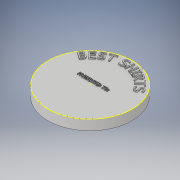
# Autodesk Inventor part: Best Shirts
Saved by Autodesk Inventor 2018.2 (Build 222227000, 227)
## iProperties
Created: 2018-03-07
Part Number: Best Shirts
Material: Generic
Document SubType Name: Modeling
Designer: battin.michael
Density: 1 g/cm^3
Appearance: Default
Author: battin.michael
Autodesk Inventor part; units mm, degrees
ref_plane "YZ Plane" through (0, 0, 0) normal (1, 0, 0) x (0, 1, 0)
ref_plane "XZ Plane" through (0, 0, 0) normal (0, 1, 0) x (-1, 0, 0)
ref_plane "XY Plane" through (0, 0, 0) normal (0, 0, 1) x (1, 0, 0)
sketch "Sketch1" plane through (0, 0, 0) normal (0, 1, 0) x (-1, 0, 0)
  circle A0 centre (0, 0) radius 104.775
  dimension "d0" = 209.55
  constraints: 1 centre point, 1 coincident
  measures "d0" diameter of A0
extrude "Extrusion1" add sketch "Sketch1" along normal blind 25.4
sketch "Sketch2" plane through (0, 25.4, 0) normal (0, 1, 0) x (1, 0, 0)
  circle A0 centre (0, 0) radius 104.775
  spline S0 degree 2 poles (-64.2326, 55.1931) (-62.9995, 54.313) (-61.7794, 52.0259) (-61.7177, 50.8085) knots 0 0 0 1 2 2 2
  spline S1 degree 2 poles (-61.7177, 50.8085) (-61.6636, 49.3537) (-62.5681, 46.7826) (-63.7735, 45.0938) knots 0 0 0 1 2 2 2
  line L0 (-63.7735, 45.0938) -> (-67.16, 40.3492)
  line L1 (-67.16, 40.3492) -> (-83.6992, 52.1542)
  line L2 (-83.6992, 52.1542) -> (-80.571, 56.5369)
  spline S2 degree 2 poles (-80.571, 56.5369) (-79.3082, 58.3061) (-77.8176, 59.9127) (-76.8013, 60.4011) knots 0 0 0 1 2 2 2
  spline S3 degree 2 poles (-76.8013, 60.4011) (-75.6913, 60.9643) (-73.5664, 60.6818) (-72.5209, 59.9356) knots 0 0 0 1 2 2 2
  spline S4 degree 2 poles (-72.5209, 59.9356) (-71.3549, 59.1033) (-70.3854, 56.5501) (-70.6376, 55.0913) knots 0 0 0 1 2 2 2
  line L3 (-70.6376, 55.0913) -> (-70.5571, 55.0339)
  spline S5 degree 2 poles (-70.5571, 55.0339) (-69.1027, 56.2213) (-65.8141, 56.322) (-64.2326, 55.1931) knots 0 0 0 1 2 2 2
  spline S6 degree 2 poles (-65.7746, 52.8343) (-66.7128, 53.5039) (-68.3018, 53.8288) (-69.3046, 53.3307) knots 0 0 0 1 2 2 2
  spline S7 degree 2 poles (-69.3046, 53.3307) (-69.9458, 52.9993) (-70.9867, 51.8811) (-71.7999, 50.7418) knots 0 0 0 1 2 2 2
  line L4 (-71.7999, 50.7418) -> (-73.5792, 48.2489)
  line L5 (-73.5792, 48.2489) -> (-67.4675, 43.8866)
  line L6 (-67.4675, 43.8866) -> (-66.1952, 45.6692)
  spline S8 degree 2 poles (-66.1952, 45.6692) (-65.162, 47.1167) (-64.2438, 48.97) (-64.2135, 49.9194) knots 0 0 0 1 2 2 2
  spline S9 degree 2 poles (-64.2135, 49.9194) (-64.2158, 50.8517) (-64.9034, 52.2124) (-65.7746, 52.8343) knots 0 0 0 1 2 2 2
  spline S10 degree 2 poles (-73.8485, 57.4237) (-74.4383, 57.8446) (-75.6098, 58.0739) (-76.1802, 57.8133) knots 0 0 0 1 2 2 2
  spline S11 degree 2 poles (-76.1802, 57.8133) (-76.8577, 57.4877) (-77.9197, 56.2833) (-78.752, 55.1172) knots 0 0 0 1 2 2 2
  line L7 (-78.752, 55.1172) -> (-80.2539, 53.0129)
  line L8 (-80.2539, 53.0129) -> (-75.4154, 49.5595)
  line L9 (-75.4154, 49.5595) -> (-73.6361, 52.0524)
  spline S12 degree 2 poles (-73.6361, 52.0524) (-72.8995, 53.0844) (-72.4156, 54.2159) (-72.3775, 54.9778) knots 0 0 0 1 2 2 2
  spline S13 degree 2 poles (-72.3775, 54.9778) (-72.3357, 55.7167) (-73.0712, 56.8688) (-73.8485, 57.4237) knots 0 0 0 1 2 2 2
  line L10 (-57.2472, 53.4467) -> (-71.0363, 68.372)
  line L11 (-71.0363, 68.372) -> (-61.699, 76.9986)
  line L12 (-61.699, 76.9986) -> (-60.0675, 75.2327)
  line L13 (-60.0675, 75.2327) -> (-67.4213, 68.4387)
  line L14 (-67.4213, 68.4387) -> (-63.6444, 64.3506)
  line L15 (-63.6444, 64.3506) -> (-56.7865, 70.6864)
  line L16 (-56.7865, 70.6864) -> (-55.155, 68.9205)
  line L17 (-55.155, 68.9205) -> (-62.0129, 62.5847)
  line L18 (-62.0129, 62.5847) -> (-56.8951, 57.0452)
  line L19 (-56.8951, 57.0452) -> (-49.5413, 63.8392)
  line L20 (-49.5413, 63.8392) -> (-47.9099, 62.0733)
  line L21 (-47.9099, 62.0733) -> (-57.2472, 53.4467)
  spline S14 degree 2 poles (-40.455, 66.3877) (-42.3401, 65.2409) (-45.4642, 64.4197) (-46.9742, 64.2721) knots 0 0 0 1 2 2 2
  line L22 (-46.9742, 64.2721) -> (-48.7372, 67.1701)
  line L23 (-48.7372, 67.1701) -> (-48.5684, 67.2728)
  spline S15 degree 2 poles (-48.5684, 67.2728) (-46.7784, 66.8969) (-43.1756, 67.4696) (-41.8391, 68.2827) knots 0 0 0 1 2 2 2
  spline S16 degree 2 poles (-41.8391, 68.2827) (-39.9259, 69.4466) (-38.9375, 72.2259) (-39.7334, 73.5342) knots 0 0 0 1 2 2 2
  spline S17 degree 2 poles (-39.7334, 73.5342) (-40.3668, 74.5753) (-42.1811, 75.2448) (-43.4893, 74.8922) knots 0 0 0 1 2 2 2
  spline S18 degree 2 poles (-43.4893, 74.8922) (-44.4281, 74.6295) (-45.9529, 74.1259) (-47.1058, 73.7715) knots 0 0 0 1 2 2 2
  spline S19 degree 2 poles (-47.1058, 73.7715) (-48.1516, 73.4629) (-50.0089, 73.316) (-50.9085, 73.559) knots 0 0 0 1 2 2 2
  spline S20 degree 2 poles (-50.9085, 73.559) (-51.794, 73.8106) (-53.3262, 74.9986) (-53.9425, 76.0115) knots 0 0 0 1 2 2 2
  spline S21 degree 2 poles (-53.9425, 76.0115) (-55.2262, 78.1217) (-53.6717, 82.9801) (-51.1253, 84.5292) knots 0 0 0 1 2 2 2
  spline S22 degree 2 poles (-51.1253, 84.5292) (-49.6623, 85.4193) (-46.7229, 86.4172) (-45.2777, 86.5447) knots 0 0 0 1 2 2 2
  line L24 (-45.2777, 86.5447) -> (-43.6003, 83.7874)
  line L25 (-43.6003, 83.7874) -> (-43.7691, 83.6847)
  spline S23 degree 2 poles (-43.7691, 83.6847) (-45.0613, 83.9394) (-48.3344, 83.4901) (-49.7553, 82.6257) knots 0 0 0 1 2 2 2
  spline S24 degree 2 poles (-49.7553, 82.6257) (-51.3591, 81.65) (-52.4269, 78.938) (-51.6823, 77.7141) knots 0 0 0 1 2 2 2
  spline S25 degree 2 poles (-51.6823, 77.7141) (-51.0148, 76.6168) (-49.0512, 76.0188) (-47.7742, 76.391) knots 0 0 0 1 2 2 2
  spline S26 degree 2 poles (-47.7742, 76.391) (-46.9228, 76.6391) (-44.4904, 77.4249) (-43.6587, 77.6418) knots 0 0 0 1 2 2 2
  spline S27 degree 2 poles (-43.6587, 77.6418) (-41.5382, 78.1801) (-38.5346, 76.9813) (-37.5503, 75.3635) knots 0 0 0 1 2 2 2
  spline S28 degree 2 poles (-37.5503, 75.3635) (-36.9256, 74.3365) (-36.5574, 71.8621) (-36.8837, 70.7191) knots 0 0 0 1 2 2 2
  spline S29 degree 2 poles (-36.8837, 70.7191) (-37.2515, 69.4545) (-38.8653, 67.3548) (-40.455, 66.3877) knots 0 0 0 1 2 2 2
  line L26 (-27.5594, 73.094) -> (-33.5858, 89.9659)
  line L27 (-33.5858, 89.9659) -> (-40.0058, 87.6728)
  line L28 (-40.0058, 87.6728) -> (-40.8145, 89.9368)
  line L29 (-40.8145, 89.9368) -> (-25.4313, 95.4315)
  line L30 (-25.4313, 95.4315) -> (-24.6226, 93.1674)
  line L31 (-24.6226, 93.1674) -> (-31.0426, 90.8743)
  line L32 (-31.0426, 90.8743) -> (-25.0162, 74.0024)
  line L33 (-25.0162, 74.0024) -> (-27.5594, 73.094)
  spline S30 degree 2 poles (-2.2308, 77.7107) (-4.4365, 77.6491) (-7.5568, 78.4843) (-8.9414, 79.1045) knots 0 0 0 1 2 2 2
  line L34 (-8.9414, 79.1045) -> (-9.0363, 82.4953)
  line L35 (-9.0363, 82.4953) -> (-8.8387, 82.5009)
  spline S31 degree 2 poles (-8.8387, 82.5009) (-7.4705, 81.2872) (-4.0574, 79.9989) (-2.4937, 80.0426) knots 0 0 0 1 2 2 2
  spline S32 degree 2 poles (-2.4937, 80.0426) (-0.2551, 80.1052) (1.9809, 82.0292) (1.9381, 83.56) knots 0 0 0 1 2 2 2
  spline S33 degree 2 poles (1.9381, 83.56) (1.904, 84.7781) (0.6601, 86.2588) (-0.6509, 86.601) knots 0 0 0 1 2 2 2
  spline S34 degree 2 poles (-0.6509, 86.601) (-1.5965, 86.8382) (-3.1704, 87.1566) (-4.3473, 87.4202) knots 0 0 0 1 2 2 2
  spline S35 degree 2 poles (-4.3473, 87.4202) (-5.4086, 87.6705) (-7.0946, 88.4635) (-7.7554, 89.1204) knots 0 0 0 1 2 2 2
  spline S36 degree 2 poles (-7.7554, 89.1204) (-8.3998, 89.7778) (-9.1417, 91.5691) (-9.1749, 92.7543) knots 0 0 0 1 2 2 2
  spline S37 degree 2 poles (-9.1749, 92.7543) (-9.2439, 95.2233) (-5.4856, 98.6725) (-2.5063, 98.7558) knots 0 0 0 1 2 2 2
  spline S38 degree 2 poles (-2.5063, 98.7558) (-0.7945, 98.8037) (2.2531, 98.2135) (3.5714, 97.6079) knots 0 0 0 1 2 2 2
  line L36 (3.5714, 97.6079) -> (3.6617, 94.3817)
  line L37 (3.6617, 94.3817) -> (3.4641, 94.3762)
  spline S39 degree 2 poles (3.4641, 94.3762) (2.4681, 95.2379) (-0.5974, 96.47) (-2.2599, 96.4235) knots 0 0 0 1 2 2 2
  spline S40 degree 2 poles (-2.2599, 96.4235) (-4.1364, 96.371) (-6.408, 94.5449) (-6.368, 93.1128) knots 0 0 0 1 2 2 2
  spline S41 degree 2 poles (-6.368, 93.1128) (-6.3321, 91.8289) (-4.9231, 90.3363) (-3.6295, 90.0265) knots 0 0 0 1 2 2 2
  spline S42 degree 2 poles (-3.6295, 90.0265) (-2.7671, 89.82) (-0.265, 89.297) (0.5649, 89.0731) knots 0 0 0 1 2 2 2
  spline S43 degree 2 poles (0.5649, 89.0731) (2.6733, 88.4896) (4.6879, 85.9596) (4.7408, 84.0667) knots 0 0 0 1 2 2 2
  spline S44 degree 2 poles (4.7408, 84.0667) (4.7744, 82.8651) (3.8677, 80.5335) (3.0179, 79.7025) knots 0 0 0 1 2 2 2
  spline S45 degree 2 poles (3.0179, 79.7025) (2.0716, 78.7865) (-0.3708, 77.7628) (-2.2308, 77.7107) knots 0 0 0 1 2 2 2
  line L38 (22.1122, 75.2719) -> (19.461, 75.7861)
  line L39 (19.461, 75.7861) -> (21.3546, 85.5501)
  line L40 (21.3546, 85.5501) -> (12.1725, 87.3308)
  line L41 (12.1725, 87.3308) -> (10.279, 77.5668)
  line L42 (10.279, 77.5668) -> (7.6278, 78.0809)
  line L43 (7.6278, 78.0809) -> (11.4964, 98.0293)
  line L44 (11.4964, 98.0293) -> (14.1476, 97.5151)
  line L45 (14.1476, 97.5151) -> (12.6302, 89.691)
  line L46 (12.6302, 89.691) -> (21.8123, 87.9103)
  line L47 (21.8123, 87.9103) -> (23.3296, 95.7344)
  line L48 (23.3296, 95.7344) -> (25.9808, 95.2203)
  line L49 (25.9808, 95.2203) -> (22.1122, 75.2719)
  line L50 (32.5045, 71.1286) -> (25.1902, 74.0365)
  line L51 (25.1902, 74.0365) -> (25.9567, 75.9645)
  line L52 (25.9567, 75.9645) -> (28.3591, 75.0094)
  line L53 (28.3591, 75.0094) -> (34.3331, 90.0358)
  line L54 (34.3331, 90.0358) -> (31.9307, 90.9909)
  line L55 (31.9307, 90.9909) -> (32.6972, 92.9189)
  line L56 (32.6972, 92.9189) -> (40.0115, 90.011)
  line L57 (40.0115, 90.011) -> (39.245, 88.083)
  line L58 (39.245, 88.083) -> (36.8426, 89.0381)
  line L59 (36.8426, 89.0381) -> (30.8686, 74.0117)
  line L60 (30.8686, 74.0117) -> (33.271, 73.0566)
  line L61 (33.271, 73.0566) -> (32.5045, 71.1286)
  line L62 (48.939, 61.5502) -> (45.9592, 63.4002)
  line L63 (45.9592, 63.4002) -> (44.7675, 73.6565)
  line L64 (44.7675, 73.6565) -> (42.1373, 75.2894)
  line L65 (42.1373, 75.2894) -> (37.8729, 68.4202)
  line L66 (37.8729, 68.4202) -> (35.5785, 69.8446)
  line L67 (35.5785, 69.8446) -> (46.2961, 87.1084)
  line L68 (46.2961, 87.1084) -> (50.7449, 84.3465)
  spline S46 degree 2 poles (50.7449, 84.3465) (52.2279, 83.4258) (54.0287, 81.8621) (54.5732, 80.71) knots 0 0 0 1 2 2 2
  spline S47 degree 2 poles (54.5732, 80.71) (55.1178, 79.5578) (55.0293, 77.0737) (54.1869, 75.7167) knots 0 0 0 1 2 2 2
  spline S48 degree 2 poles (54.1869, 75.7167) (53.0144, 73.8281) (49.4943, 72.4664) (47.4614, 72.8757) knots 0 0 0 1 2 2 2
  line L69 (47.4614, 72.8757) -> (48.939, 61.5502)
  spline S49 degree 2 poles (51.6816, 77.02) (52.1506, 77.7755) (52.3399, 79.2667) (52.0148, 79.9918) knots 0 0 0 1 2 2 2
  spline S50 degree 2 poles (52.0148, 79.9918) (51.7249, 80.6176) (50.5888, 81.6911) (49.6375, 82.2817) knots 0 0 0 1 2 2 2
  line L70 (49.6375, 82.2817) -> (47.3571, 83.6974)
  line L71 (47.3571, 83.6974) -> (43.3272, 77.206)
  line L72 (43.3272, 77.206) -> (45.3418, 75.9553)
  spline S51 degree 2 poles (45.3418, 75.9553) (46.3351, 75.3387) (48.1331, 74.707) (49.0174, 74.9139) knots 0 0 0 1 2 2 2
  spline S52 degree 2 poles (49.0174, 74.9139) (49.8163, 75.0769) (51.1258, 76.1246) (51.6816, 77.02) knots 0 0 0 1 2 2 2
  line L73 (53.4089, 57.0066) -> (65.8849, 69.8645)
  line L74 (65.8849, 69.8645) -> (60.9922, 74.6118)
  line L75 (60.9922, 74.6118) -> (62.6664, 76.3373)
  line L76 (62.6664, 76.3373) -> (74.3898, 64.9621)
  line L77 (74.3898, 64.9621) -> (72.7157, 63.2367)
  line L78 (72.7157, 63.2367) -> (67.823, 67.984)
  line L79 (67.823, 67.984) -> (55.347, 55.126)
  line L80 (55.347, 55.126) -> (53.4089, 57.0066)
  spline S53 degree 2 poles (64.2632, 43.7513) (63.0228, 45.5762) (62.0451, 48.6549) (61.8215, 50.1555) knots 0 0 0 1 2 2 2
  line L81 (61.8215, 50.1555) -> (64.6269, 52.0624)
  line L82 (64.6269, 52.0624) -> (64.738, 51.899)
  spline S54 degree 2 poles (64.738, 51.899) (64.4528, 50.0923) (65.2065, 46.523) (66.086, 45.2292) knots 0 0 0 1 2 2 2
  spline S55 degree 2 poles (66.086, 45.2292) (67.3449, 43.3771) (70.1705, 42.5301) (71.437, 43.391) knots 0 0 0 1 2 2 2
  spline S56 degree 2 poles (71.437, 43.391) (72.4448, 44.076) (73.0219, 45.9218) (72.6039, 47.2106) knots 0 0 0 1 2 2 2
  spline S57 degree 2 poles (72.6039, 47.2106) (72.2941, 48.135) (71.7143, 49.6324) (71.3022, 50.7659) knots 0 0 0 1 2 2 2
  spline S58 degree 2 poles (71.3022, 50.7659) (70.9413, 51.7949) (70.7009, 53.6425) (70.8982, 54.5531) knots 0 0 0 1 2 2 2
  spline S59 degree 2 poles (70.8982, 54.5531) (71.1048, 55.4501) (72.2141, 57.0404) (73.1946, 57.7069) knots 0 0 0 1 2 2 2
  spline S60 degree 2 poles (73.1946, 57.7069) (75.2374, 59.0954) (80.1681, 57.7878) (81.8436, 55.3229) knots 0 0 0 1 2 2 2
  spline S61 degree 2 poles (81.8436, 55.3229) (82.8063, 53.9066) (83.9512, 51.0212) (84.1514, 49.5843) knots 0 0 0 1 2 2 2
  line L83 (84.1514, 49.5843) -> (81.4821, 47.77)
  line L84 (81.4821, 47.77) -> (81.3711, 47.9334)
  spline S62 degree 2 poles (81.3711, 47.9334) (81.5603, 49.2368) (80.9465, 52.4831) (80.0116, 53.8586) knots 0 0 0 1 2 2 2
  spline S63 degree 2 poles (80.0116, 53.8586) (78.9563, 55.4111) (76.1939, 56.3408) (75.009, 55.5355) knots 0 0 0 1 2 2 2
  spline S64 degree 2 poles (75.009, 55.5355) (73.9468, 54.8134) (73.4486, 52.8222) (73.8847, 51.5656) knots 0 0 0 1 2 2 2
  spline S65 degree 2 poles (73.8847, 51.5656) (74.1754, 50.7278) (75.0829, 48.3382) (75.3414, 47.5184) knots 0 0 0 1 2 2 2
  spline S66 degree 2 poles (75.3414, 47.5184) (75.986, 45.4278) (74.9402, 42.3675) (73.374, 41.3029) knots 0 0 0 1 2 2 2
  spline S67 degree 2 poles (73.374, 41.3029) (72.3799, 40.6272) (69.9271, 40.1347) (68.7692, 40.4029) knots 0 0 0 1 2 2 2
  spline S68 degree 2 poles (68.7692, 40.4029) (67.4876, 40.7065) (65.3092, 42.2124) (64.2632, 43.7513) knots 0 0 0 1 2 2 2
  constraints: 1 centre point, 1 coincident, 1 other
extrude "Extrusion2" add sketch "Sketch2" along normal blind 5.08 contours S0 S1 L0 L1 L2 S2 S3 S4 L3 S5 | L10 L11 L12 L13 L14 L15 L16 L17 L18 L19 L20 L21 | S14 L22 L23 S15 S16 S17 S18 S19 S20 S21 S22 L24 L25 S23 S24 S25 S26 S27 S28 S29 | L26 L27 L28 L29 L30 L31 L32 L33 | S30 L34 L35 S31 S32 S33 S34 S35 S36 S37 S38 L36 L37 S39 S40 S41 S42 S43 S44 S45 | L38 L39 L40 L41 L42 L43 L44 L45 L46 L47 L48 L49 | L50 L51 L52 L53 L54 L55 L56 L57 L58 L59 L60 L61 | L62 L63 L64 L65 L66 L67 L68 S46 S47 S48 L69 | L73 L74 L75 L76 L77 L78 L79 L80 | S53 L81 L82 S54 S55 S56 S57 S58 S59 S60 S61 L83 L84 S62 S63 S64 S65 S66 S67 S68
sketch "Sketch3" plane through (0, 25.4, 0) normal (0, 1, 0) x (1, 0, 0)
  circle A0 centre (0, 0) radius 104.775
  constraints: 1 centre point, 1 coincident
extrude "Extrusion3" add sketch "Sketch3" along normal blind 2.54
sketch "Sketch4" plane through (0, 0, 0) normal (0, -1, 0) x (1, 0, 0)
  circle A0 centre (0, 0) radius 104.775
  constraints: 1 centre point, 1 coincident
extrude "Extrusion4" cut sketch "Sketch4" against normal blind 2.54
sketch "Sketch5" plane through (0, 27.94, 0) normal (0, 1, 0) x (1, 0, 0)
  circle A0 centre (0, 0) radius 104.775 projected
  circle A1 centre (0, 0) radius 104.775 projected
sketch "Sketch6" plane through (0, 27.94, 0) normal (0, 1, 0) x (1, 0, 0)
  circle A0 centre (0, 0) radius 104.775 projected
  spline S0 degree 2 poles (-32.6567, 10.8618) (-32.6567, 10.3678) (-33.0087, 9.4786) (-33.3236, 9.1698) knots 0 0 0 1 2 2 2
  spline S1 degree 2 poles (-33.3236, 9.1698) (-33.7188, 8.7808) (-34.7871, 8.3794) (-35.6022, 8.3794) knots 0 0 0 1 2 2 2
  line L0 (-35.6022, 8.3794) -> (-36.4605, 8.3794)
  line L1 (-36.4605, 8.3794) -> (-36.4605, 5.5389)
  line L2 (-36.4605, 5.5389) -> (-37.4732, 5.5389)
  line L3 (-37.4732, 5.5389) -> (-37.4732, 13.1589)
  line L4 (-37.4732, 13.1589) -> (-35.559, 13.1589)
  spline S2 degree 2 poles (-35.559, 13.1589) (-34.8797, 13.1589) (-33.9288, 12.9366) (-33.5644, 12.6834) knots 0 0 0 1 2 2 2
  spline S3 degree 2 poles (-33.5644, 12.6834) (-33.1384, 12.3932) (-32.6567, 11.4978) (-32.6567, 10.8618) knots 0 0 0 1 2 2 2
  spline S4 degree 2 poles (-33.7126, 10.8309) (-33.7126, 11.2261) (-33.9843, 11.8066) (-34.2622, 11.9918) knots 0 0 0 1 2 2 2
  spline S5 degree 2 poles (-34.2622, 11.9918) (-34.503, 12.1524) (-35.1452, 12.2821) (-35.6207, 12.2821) knots 0 0 0 1 2 2 2
  line L5 (-35.6207, 12.2821) -> (-36.4605, 12.2821)
  line L6 (-36.4605, 12.2821) -> (-36.4605, 9.2439)
  line L7 (-36.4605, 9.2439) -> (-35.7689, 9.2439)
  spline S6 degree 2 poles (-35.7689, 9.2439) (-35.1514, 9.2439) (-34.3919, 9.4415) (-34.1449, 9.7009) knots 0 0 0 1 2 2 2
  spline S7 degree 2 poles (-34.1449, 9.7009) (-33.9164, 9.9294) (-33.7126, 10.4666) (-33.7126, 10.8309) knots 0 0 0 1 2 2 2
  line L8 (-25.7962, 5.5389) -> (-27.1115, 5.5389)
  line L9 (-27.1115, 5.5389) -> (-29.5198, 8.5709)
  line L10 (-29.5198, 8.5709) -> (-30.6807, 8.5709)
  line L11 (-30.6807, 8.5709) -> (-30.6807, 5.5389)
  line L12 (-30.6807, 5.5389) -> (-31.6934, 5.5389)
  line L13 (-31.6934, 5.5389) -> (-31.6934, 13.1589)
  line L14 (-31.6934, 13.1589) -> (-29.7297, 13.1589)
  spline S8 degree 2 poles (-29.7297, 13.1589) (-29.0752, 13.1589) (-28.1921, 13.0169) (-27.7908, 12.7575) knots 0 0 0 1 2 2 2
  spline S9 degree 2 poles (-27.7908, 12.7575) (-27.3894, 12.4982) (-26.9263, 11.6893) (-26.9263, 11.0903) knots 0 0 0 1 2 2 2
  spline S10 degree 2 poles (-26.9263, 11.0903) (-26.9263, 10.2567) (-27.7784, 9.1266) (-28.5071, 8.8549) knots 0 0 0 1 2 2 2
  line L15 (-28.5071, 8.8549) -> (-25.7962, 5.5389)
  spline S11 degree 2 poles (-27.9822, 11.01) (-27.9822, 11.3435) (-28.2168, 11.856) (-28.4638, 12.0227) knots 0 0 0 1 2 2 2
  spline S12 degree 2 poles (-28.4638, 12.0227) (-28.68, 12.1647) (-29.2543, 12.2821) (-29.6742, 12.2821) knots 0 0 0 1 2 2 2
  line L16 (-29.6742, 12.2821) -> (-30.6807, 12.2821)
  line L17 (-30.6807, 12.2821) -> (-30.6807, 9.4168)
  line L18 (-30.6807, 9.4168) -> (-29.7915, 9.4168)
  spline S13 degree 2 poles (-29.7915, 9.4168) (-29.3531, 9.4168) (-28.6553, 9.5712) (-28.4144, 9.8121) knots 0 0 0 1 2 2 2
  spline S14 degree 2 poles (-28.4144, 9.8121) (-28.1921, 10.022) (-27.9822, 10.6148) (-27.9822, 11.01) knots 0 0 0 1 2 2 2
  line L19 (-25.1911, 5.5389) -> (-25.1911, 13.1589)
  line L20 (-25.1911, 13.1589) -> (-20.4239, 13.1589)
  line L21 (-20.4239, 13.1589) -> (-20.4239, 12.2574)
  line L22 (-20.4239, 12.2574) -> (-24.1784, 12.2574)
  line L23 (-24.1784, 12.2574) -> (-24.1784, 10.1702)
  line L24 (-24.1784, 10.1702) -> (-20.6771, 10.1702)
  line L25 (-20.6771, 10.1702) -> (-20.6771, 9.2686)
  line L26 (-20.6771, 9.2686) -> (-24.1784, 9.2686)
  line L27 (-24.1784, 9.2686) -> (-24.1784, 6.4405)
  line L28 (-24.1784, 6.4405) -> (-20.4239, 6.4405)
  line L29 (-20.4239, 6.4405) -> (-20.4239, 5.5389)
  line L30 (-20.4239, 5.5389) -> (-25.1911, 5.5389)
  spline S15 degree 2 poles (-17.1882, 5.4031) (-18.0157, 5.4031) (-19.1766, 5.7489) (-19.6891, 5.9959) knots 0 0 0 1 2 2 2
  line L31 (-19.6891, 5.9959) -> (-19.6891, 7.2679)
  line L32 (-19.6891, 7.2679) -> (-19.615, 7.2679)
  spline S16 degree 2 poles (-19.615, 7.2679) (-19.1148, 6.7986) (-17.849, 6.2799) (-17.2623, 6.2799) knots 0 0 0 1 2 2 2
  spline S17 degree 2 poles (-17.2623, 6.2799) (-16.4225, 6.2799) (-15.5642, 6.9777) (-15.5642, 7.552) knots 0 0 0 1 2 2 2
  spline S18 degree 2 poles (-15.5642, 7.552) (-15.5642, 8.0089) (-16.015, 8.577) (-16.5028, 8.7191) knots 0 0 0 1 2 2 2
  spline S19 degree 2 poles (-16.5028, 8.7191) (-16.8548, 8.8179) (-17.4414, 8.9537) (-17.8798, 9.0649) knots 0 0 0 1 2 2 2
  spline S20 degree 2 poles (-17.8798, 9.0649) (-18.275, 9.1698) (-18.8987, 9.4848) (-19.1395, 9.738) knots 0 0 0 1 2 2 2
  spline S21 degree 2 poles (-19.1395, 9.738) (-19.3742, 9.9911) (-19.6335, 10.6704) (-19.6335, 11.115) knots 0 0 0 1 2 2 2
  spline S22 degree 2 poles (-19.6335, 11.115) (-19.6335, 12.0412) (-18.1886, 13.2948) (-17.0709, 13.2948) knots 0 0 0 1 2 2 2
  spline S23 degree 2 poles (-17.0709, 13.2948) (-16.4287, 13.2948) (-15.2925, 13.0416) (-14.8047, 12.8008) knots 0 0 0 1 2 2 2
  line L33 (-14.8047, 12.8008) -> (-14.8047, 11.5905)
  line L34 (-14.8047, 11.5905) -> (-14.8788, 11.5905)
  spline S24 degree 2 poles (-14.8788, 11.5905) (-15.2431, 11.9239) (-16.3793, 12.4179) (-17.003, 12.4179) knots 0 0 0 1 2 2 2
  spline S25 degree 2 poles (-17.003, 12.4179) (-17.7069, 12.4179) (-18.5776, 11.7572) (-18.5776, 11.22) knots 0 0 0 1 2 2 2
  spline S26 degree 2 poles (-18.5776, 11.22) (-18.5776, 10.7383) (-18.0651, 10.164) (-17.5834, 10.0344) knots 0 0 0 1 2 2 2
  spline S27 degree 2 poles (-17.5834, 10.0344) (-17.2623, 9.9479) (-16.3299, 9.7256) (-16.0211, 9.633) knots 0 0 0 1 2 2 2
  spline S28 degree 2 poles (-16.0211, 9.633) (-15.2369, 9.3921) (-14.5083, 8.4227) (-14.5083, 7.7125) knots 0 0 0 1 2 2 2
  spline S29 degree 2 poles (-14.5083, 7.7125) (-14.5083, 7.2618) (-14.8726, 6.3973) (-15.1999, 6.0947) knots 0 0 0 1 2 2 2
  spline S30 degree 2 poles (-15.1999, 6.0947) (-15.5642, 5.7612) (-16.4904, 5.4031) (-17.1882, 5.4031) knots 0 0 0 1 2 2 2
  line L35 (-13.477, 5.5389) -> (-13.477, 13.1589)
  line L36 (-13.477, 13.1589) -> (-8.7099, 13.1589)
  line L37 (-8.7099, 13.1589) -> (-8.7099, 12.2574)
  line L38 (-8.7099, 12.2574) -> (-12.4643, 12.2574)
  line L39 (-12.4643, 12.2574) -> (-12.4643, 10.1702)
  line L40 (-12.4643, 10.1702) -> (-8.9631, 10.1702)
  line L41 (-8.9631, 10.1702) -> (-8.9631, 9.2686)
  line L42 (-8.9631, 9.2686) -> (-12.4643, 9.2686)
  line L43 (-12.4643, 9.2686) -> (-12.4643, 6.4405)
  line L44 (-12.4643, 6.4405) -> (-8.7099, 6.4405)
  line L45 (-8.7099, 6.4405) -> (-8.7099, 5.5389)
  line L46 (-8.7099, 5.5389) -> (-13.477, 5.5389)
  line L47 (-2.1458, 5.5389) -> (-3.282, 5.5389)
  line L48 (-3.282, 5.5389) -> (-6.6536, 12.1092)
  line L49 (-6.6536, 12.1092) -> (-6.6536, 5.5389)
  line L50 (-6.6536, 5.5389) -> (-7.5984, 5.5389)
  line L51 (-7.5984, 5.5389) -> (-7.5984, 13.1589)
  line L52 (-7.5984, 13.1589) -> (-6.1596, 13.1589)
  line L53 (-6.1596, 13.1589) -> (-3.0906, 7.1259)
  line L54 (-3.0906, 7.1259) -> (-3.0906, 13.1589)
  line L55 (-3.0906, 13.1589) -> (-2.1458, 13.1589)
  line L56 (-2.1458, 13.1589) -> (-2.1458, 5.5389)
  line L57 (1.1763, 5.5389) -> (1.1763, 12.2574)
  line L58 (1.1763, 12.2574) -> (-1.3801, 12.2574)
  line L59 (-1.3801, 12.2574) -> (-1.3801, 13.1589)
  line L60 (-1.3801, 13.1589) -> (4.7455, 13.1589)
  line L61 (4.7455, 13.1589) -> (4.7455, 12.2574)
  line L62 (4.7455, 12.2574) -> (2.1891, 12.2574)
  line L63 (2.1891, 12.2574) -> (2.1891, 5.5389)
  line L64 (2.1891, 5.5389) -> (1.1763, 5.5389)
  line L65 (5.5174, 5.5389) -> (5.5174, 13.1589)
  line L66 (5.5174, 13.1589) -> (10.2845, 13.1589)
  line L67 (10.2845, 13.1589) -> (10.2845, 12.2574)
  line L68 (10.2845, 12.2574) -> (6.5301, 12.2574)
  line L69 (6.5301, 12.2574) -> (6.5301, 10.1702)
  line L70 (6.5301, 10.1702) -> (10.0314, 10.1702)
  line L71 (10.0314, 10.1702) -> (10.0314, 9.2686)
  line L72 (10.0314, 9.2686) -> (6.5301, 9.2686)
  line L73 (6.5301, 9.2686) -> (6.5301, 6.4405)
  line L74 (6.5301, 6.4405) -> (10.2845, 6.4405)
  line L75 (10.2845, 6.4405) -> (10.2845, 5.5389)
  line L76 (10.2845, 5.5389) -> (5.5174, 5.5389)
  spline S31 degree 2 poles (17.4044, 9.3427) (17.4044, 8.2992) (16.5584, 6.6196) (15.8482, 6.1503) knots 0 0 0 1 2 2 2
  spline S32 degree 2 poles (15.8482, 6.1503) (15.2678, 5.7859) (14.076, 5.5389) (13.1498, 5.5389) knots 0 0 0 1 2 2 2
  line L77 (13.1498, 5.5389) -> (11.396, 5.5389)
  line L78 (11.396, 5.5389) -> (11.396, 13.1589)
  line L79 (11.396, 13.1589) -> (13.1312, 13.1589)
  spline S33 degree 2 poles (13.1312, 13.1589) (14.2057, 13.1589) (15.4283, 12.8378) (15.8606, 12.5538) knots 0 0 0 1 2 2 2
  spline S34 degree 2 poles (15.8606, 12.5538) (16.5954, 12.0659) (17.4044, 10.4543) (17.4044, 9.3427) knots 0 0 0 1 2 2 2
  spline S35 degree 2 poles (16.3484, 9.3551) (16.3484, 10.232) (15.768, 11.4731) (15.1937, 11.8251) knots 0 0 0 1 2 2 2
  spline S36 degree 2 poles (15.1937, 11.8251) (14.7861, 12.0659) (13.8661, 12.2821) (13.1806, 12.2821) knots 0 0 0 1 2 2 2
  line L80 (13.1806, 12.2821) -> (12.4087, 12.2821)
  line L81 (12.4087, 12.2821) -> (12.4087, 6.4158)
  line L82 (12.4087, 6.4158) -> (13.1806, 6.4158)
  spline S37 degree 2 poles (13.1806, 6.4158) (13.8537, 6.4158) (14.8726, 6.6319) (15.2863, 6.9221) knots 0 0 0 1 2 2 2
  spline S38 degree 2 poles (15.2863, 6.9221) (15.8174, 7.2803) (16.3484, 8.4659) (16.3484, 9.3551) knots 0 0 0 1 2 2 2
  line L83 (23.5547, 5.5389) -> (23.5547, 12.2574)
  line L84 (23.5547, 12.2574) -> (20.9982, 12.2574)
  line L85 (20.9982, 12.2574) -> (20.9982, 13.1589)
  line L86 (20.9982, 13.1589) -> (27.1239, 13.1589)
  line L87 (27.1239, 13.1589) -> (27.1239, 12.2574)
  line L88 (27.1239, 12.2574) -> (24.5674, 12.2574)
  line L89 (24.5674, 12.2574) -> (24.5674, 5.5389)
  line L90 (24.5674, 5.5389) -> (23.5547, 5.5389)
  spline S39 degree 2 poles (33.2866, 12.2882) (33.7188, 11.7819) (34.2005, 10.2999) (34.2005, 9.3489) knots 0 0 0 1 2 2 2
  spline S40 degree 2 poles (34.2005, 9.3489) (34.2005, 8.4227) (33.7312, 6.9221) (33.2866, 6.4158) knots 0 0 0 1 2 2 2
  spline S41 degree 2 poles (33.2866, 6.4158) (32.8173, 5.8847) (31.5761, 5.3784) (30.8289, 5.3784) knots 0 0 0 1 2 2 2
  spline S42 degree 2 poles (30.8289, 5.3784) (30.057, 5.3784) (28.822, 5.9033) (28.3712, 6.4158) knots 0 0 0 1 2 2 2
  spline S43 degree 2 poles (28.3712, 6.4158) (27.9328, 6.9221) (27.4635, 8.4103) (27.4635, 9.3489) knots 0 0 0 1 2 2 2
  spline S44 degree 2 poles (27.4635, 9.3489) (27.4635, 10.3061) (27.939, 11.7634) (28.3774, 12.2882) knots 0 0 0 1 2 2 2
  spline S45 degree 2 poles (28.3774, 12.2882) (28.822, 12.7946) (30.0632, 13.3195) (30.8289, 13.3195) knots 0 0 0 1 2 2 2
  spline S46 degree 2 poles (30.8289, 13.3195) (31.6069, 13.3195) (32.8543, 12.7761) (33.2866, 12.2882) knots 0 0 0 1 2 2 2
  spline S47 degree 2 poles (33.1445, 9.3489) (33.1445, 10.1023) (32.8173, 11.2694) (32.5209, 11.6522) knots 0 0 0 1 2 2 2
  spline S48 degree 2 poles (32.5209, 11.6522) (32.2183, 12.0474) (31.3661, 12.4426) (30.8351, 12.4426) knots 0 0 0 1 2 2 2
  spline S49 degree 2 poles (30.8351, 12.4426) (30.2855, 12.4426) (29.458, 12.0598) (29.1431, 11.6522) knots 0 0 0 1 2 2 2
  spline S50 degree 2 poles (29.1431, 11.6522) (28.8405, 11.2632) (28.5194, 10.0899) (28.5194, 9.3489) knots 0 0 0 1 2 2 2
  spline S51 degree 2 poles (28.5194, 9.3489) (28.5194, 7.8484) (29.7791, 6.2552) (30.8351, 6.2552) knots 0 0 0 1 2 2 2
  spline S52 degree 2 poles (30.8351, 6.2552) (31.891, 6.2552) (33.1445, 7.8484) (33.1445, 9.3489) knots 0 0 0 1 2 2 2
  line L91 (37.0039, 5.5389) -> (35.7813, 5.5389)
  line L92 (35.7813, 5.5389) -> (35.7813, 6.9962)
  line L93 (35.7813, 6.9962) -> (37.0039, 6.9962)
  line L94 (37.0039, 6.9962) -> (37.0039, 5.5389)
  line L95 (37.0039, 9.7997) -> (35.7813, 9.7997)
  line L96 (35.7813, 9.7997) -> (35.7813, 11.257)
  line L97 (35.7813, 11.257) -> (37.0039, 11.257)
  line L98 (37.0039, 11.257) -> (37.0039, 9.7997)
  point P0 (-38.2451, 5.5389)
  constraints: 1 other
extrude "Extrusion5" add sketch "Sketch6" along normal blind 2.54 contours S0 S1 L0 L1 L2 L3 L4 S2 S3 | L8 L9 L10 L11 L12 L13 L14 S8 S9 S10 L15 | L19 L20 L21 L22 L23 L24 L25 L26 L27 L28 L29 L30 | S15 L31 L32 S16 S17 S18 S19 S20 S21 S22 S23 L33 L34 S24 S25 S26 S27 S28 S29 S30 | L35 L36 L37 L38 L39 L40 L41 L42 L43 L44 L45 L46 | L47 L48 L49 L50 L51 L52 L53 L54 L55 L56 | L57 L58 L59 L60 L61 L62 L63 L64 | L65 L66 L67 L68 L69 L70 L71 L72 L73 L74 L75 L76 | S31 S32 L77 L78 L79 S33 S34 | L83 L84 L85 L86 L87 L88 L89 L90 | S39 S40 S41 S42 S43 S44 S45 S46 | L91 L92 L93 L94 | L95 L96 L97 L98
sketch "Sketch7" plane through (0, 27.94, 0) normal (0, 1, 0) x (1, 0, 0)
  line L0 (-2.1458, 5.5389) -> (-3.282, 5.5389) projected
  line L1 (1.1763, 5.5389) -> (1.1763, 12.2574) projected
  point P0 (0, 0)
sketch "Sketch8" plane through (0, 27.94, 0) normal (0, 1, 0) x (1, 0, 0)
  point P0 (0, 0)
body "Solid1"
